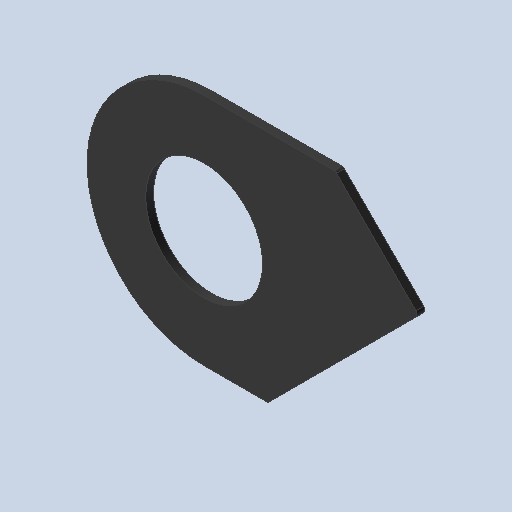
# Autodesk Inventor part: ухо
Saved by Autodesk Inventor 2026 (Build 300175000, 175)
## iProperties
Created: 2024-05-23
Part Number: ухо
Material: Generic
Document SubType Name: Sheet Metal
Designer: admin
Density: 1 g/cm^3
Flat Pattern Width: 12 cm
Flat Pattern Length: 16.9172 cm
Flat Pattern Area: 203.006 cm^2
Sheet Metal Rule: По умолчанию_мм
Sheet Metal Width: 120,000 mm
Sheet Metal Length: 169,172 mm
Sheet Metal Area: 20300,589 mm^2
Appearance: Default
Mass: 0.559799 g
Surface Area: 23.3947 cm^2
Volume: 0.559799 cm^3
Author: admin
Autodesk Inventor part; units mm, degrees
ref_plane "YZ Plane" through (0, 0, 0) normal (1, 0, 0) x (0, 1, 0)
ref_plane "XZ Plane" through (0, 0, 0) normal (0, 1, 0) x (-1, 0, 0)
ref_plane "XY Plane" through (0, 0, 0) normal (0, 0, 1) x (1, 0, 0)
sketch "Sketch1" plane through (0, 0, 0) normal (0, 0, 1) x (1, 0, 0)
  line L0 (-85, 60) -> (85, 60)
  line L1 (85, 60) -> (85, -60)
  line L2 (85, -60) -> (-85, -60)
  line L3 (-85, -60) -> (-85, 60)
  line L4 (-85, 60) -> (85, -60) construction
  line L5 (85, 60) -> (-85, -60) construction
  circle A0 centre (-25, 0) radius 30
  line L6 (0, 60) -> (0, -60) construction
  arc A1 (-25, 60) -> (-25, -60) centre (-25, 0) ccw
  line L7 (85, 17.2792) -> (7.7208, -60)
  line L8 (85, 17.2792) -> (42.2792, 60)
  point P0 (0, 0)
  point P1 (-85, 0)
  dimension "d0" = 170
  dimension "d1" = 120
  dimension "d13" = 60
  dimension "d14" = 60
  dimension "d17" = 45
  dimension "d18" = 90
  measures "d0" distance of L1.end L2.end
  measures "d1" distance of L0.end L1.end
  measures "d13" distance from line of L3 A0.centre
  measures "d14" diameter of A0
  measures "d17" angle of L2 L7
  measures "d18" distance from line of A0.centre L8
extrude "Plate1" add sketch "Sketch1" along normal blind 4 contours L0 L8 L7 L2 A1
fillet "Corner Round1" radius 2 3 edges at (85, 17.2792, 2) (42.2792, 60, 2) (7.7208, -60, 2)
equation "\"d2\" = Thickness"
equation "\"BendRadius\" = Thickness"
equation "\"BendReliefWidth\" = Thickness"
equation "\"BendReliefDepth\" = 0.5 * Thickness"
equation "\"CornerReliefSize\" = 4 * Thickness"
equation "\"MinimumRemnant\" = 2 * Thickness"
equation "\"TransitionRadius\" = BendRadius"
equation "\"JacobiRadiusSize\" = BendRadius"
equation "\"GapSize\" = Thickness"
equation "\"Thickness\" = 4"
body "Solid1"
